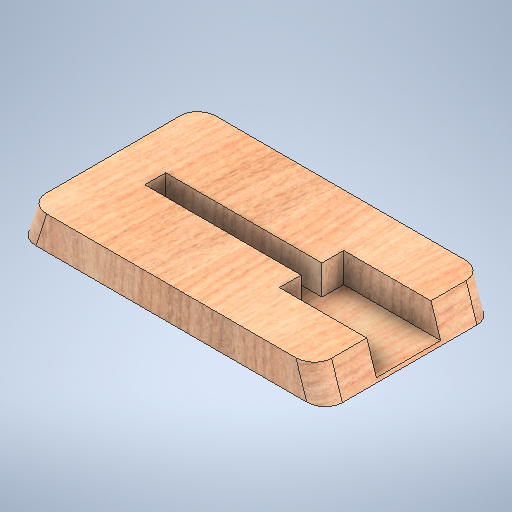
# Autodesk Inventor part: 1 part 1
Saved by Autodesk Inventor 2025.1 (Build 291241000, 241)
## iProperties
Created: 2024-07-24
Part Number: 1 part 1
Material: Holz (Birke)
Document SubType Name: Modeling
Designer: ffogue
Density: 0.55 g/cm^3
Appearance: Birke - natur - poliert
Author: ffogue
Autodesk Inventor part; units mm, degrees
ref_plane "YZ Plane" through (0, 0, 0) normal (1, 0, 0) x (0, 1, 0)
ref_plane "XZ Plane" through (0, 0, 0) normal (0, 1, 0) x (-1, 0, 0)
ref_plane "XY Plane" through (0, 0, 0) normal (0, 0, 1) x (1, 0, 0)
sketch "Skizze2" plane through (0, 0, 0) normal (0, 0, 1) x (1, 0, 0)
  line L0 (-177, 0) -> (177, 0)
  line L1 (177, 0) -> (177, 195)
  line L2 (177, 195) -> (-177, 195)
  line L3 (-177, 195) -> (-177, 0)
  point P0 (0, 0)
  point P1 (0, 0)
  dimension "d0" = 195
  dimension "d1" = 354
  constraints: 8 end point, 2 parallel, 1 coincident, 1 horizontal, 1 midpoint, 1 perpendicular
  measures "d0" distance between parallel lines of L0 L2
  measures "d1" distance between parallel lines of L1 L3
extrude "Extrusion1" add sketch "Skizze2" along normal blind 38
sketch "Skizze3" plane through (-177, 0, 0) normal (0, -1, 0) x (1, 0, 0)
  line L0 (354, 0) -> (0, 0) projected
  line L1 (0, 0) -> (15.5, 47)
  line L2 (15.5, 47) -> (0, 47)
  line L3 (0, 47) -> (0, 0)
  dimension "d7" = 15.5
  constraints: 6 end point, 1 parallel, 1 perpendicular
  measures "d7" distance of L1.end L2.end
extrude "Extrusion2" cut sketch "Skizze3" against normal up to surface (195 mm away)
mirror "Spiegeln1" about plane through (0, 0, 0) normal (1, 0, 0) of "Extrusion2"
fillet "Rundung1" radius 20 4 edges at (170.734, 0, 19) (170.734, 195, 19) (-170.734, 195, 19) (-170.734, 0, 19)
sketch "Skizze4" plane through (0, 0, 38) normal (0, 0, 1) x (1, 0, 0)
  ellipse E0 centre (-143.4086, 20) end of major axis (-164.4681, 20) minor radius 20 (-164.4681, 20) -> (-143.4086, 0) ccw projected
  line L0 (-143.4086, 0) -> (143.4086, 0) projected
  ellipse E1 centre (143.4086, 20) end of major axis (164.4681, 20) minor radius 20 (143.4086, 0) -> (164.4681, 20) ccw projected
  line L1 (164.4681, 20) -> (164.4681, 175) projected
  ellipse E2 centre (143.4086, 175) end of major axis (164.4681, 175) minor radius 20 (164.4681, 175) -> (143.4086, 195) ccw projected
  line L2 (143.4086, 195) -> (-143.4086, 195) projected
  ellipse E3 centre (-143.4086, 175) end of major axis (-164.4681, 175) minor radius 20 (-143.4086, 195) -> (-164.4681, 175) ccw projected
  line L3 (-164.4681, 175) -> (-164.4681, 20) projected
  line L4 (177, 60.5) -> (64, 60.5)
  line L5 (64, 60.5) -> (64, 85.5)
  line L6 (64, 85.5) -> (-116, 85.5)
  line L7 (-116, 85.5) -> (-116, 109.5)
  line L8 (-116, 109.5) -> (64, 109.5)
  line L9 (64, 109.5) -> (64, 134.5)
  line L10 (64, 134.5) -> (177, 134.5)
  line L11 (177, 20) -> (177, 175) projected
  line L12 (-177, 175) -> (-177, 20) projected
  line L13 (164.4681, 20) -> (164.4681, 175) projected
  point P0 (0, 0)
  point P1 (-116, 97.5)
  point P2 (164.4681, 97.5)
  point P3 (164.4681, 97.5)
  dimension "d12" = 113
  dimension "d14" = 24
  dimension "d15" = 74
  dimension "d16" = 37
  dimension "d17" = 180
  constraints: 14 end point, 5 perpendicular, 4 point on line, 3 midpoint, 1 horizontal, 1 horizontal alignment, 4 other
  measures "d12" distance of L4.start L4.end
  measures "d14" distance between parallel lines of L8 L6
  measures "d15" distance between parallel lines of L10 L4
  measures "d16" distance from line of L10 point (164.468, 97.5)
  measures "d17" distance between parallel lines of L5 L7
extrude "Extrusion3" cut sketch "Skizze4" against normal blind 34 contours L4 L5 L6 L7 L8 L9 L10 L1 | L1 L10 L11 L4
sketch "Sketch7" plane through (64, 60.5, 38) normal (1, 0, 0) x (0, 0, -1)
  line L0 (0, 25) -> (34, 25) projected
  line L1 (34, 25) -> (34, 49) projected
  line L2 (0, 49) -> (34, 49) projected
  circle A0 centre (13, 37) radius 11
  line L3 (0, 25) -> (0, 49) projected
  point P0 (38, -60.5)
  point P1 (17, 49)
  point P2 (0, 37)
  dimension "d35" = 22
  dimension "d36" = 21
  constraints: 1 centre point, 1 horizontal alignment, 1 midpoint
  measures "d35" diameter of A0
  measures "d36" distance from line of L1 A0.centre
